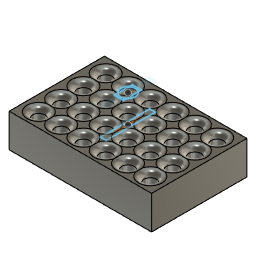
simple_rack v2 (Autodesk Fusion 360 design; units mm, degrees)
Autodesk Fusion 360 part; units mm, degrees
note: some values were not read from the file. Chosen so that the rebuilt part matches the saved one: which face or edge a step refers to. Set by a fixed rule: which sketch regions a step uses.
sketch "Sketch1" plane through (0, 0, 0) normal (0, 0, 1) x (1, 0, 0)
  circle A0 centre (0, 0) radius 5.5
  circle A1 centre (0, 0) radius 7
  circle A2 centre (20, 0) radius 7
  circle A3 centre (20, 0) radius 5.5
  circle A4 centre (40, 0) radius 7
  circle A5 centre (40, 0) radius 5.5
  circle A6 centre (60, 0) radius 7
  circle A7 centre (60, 0) radius 5.5
  circle A8 centre (80, 0) radius 7
  circle A9 centre (80, 0) radius 5.5
  circle A10 centre (100, 0) radius 7
  circle A11 centre (100, 0) radius 5.5
  circle A12 centre (0, 20) radius 7
  circle A13 centre (0, 20) radius 5.5
  circle A14 centre (20, 20) radius 7
  circle A15 centre (20, 20) radius 5.5
  circle A16 centre (40, 20) radius 7
  circle A17 centre (40, 20) radius 5.5
  circle A18 centre (60, 20) radius 7
  circle A19 centre (60, 20) radius 5.5
  circle A20 centre (80, 20) radius 7
  circle A21 centre (80, 20) radius 5.5
  circle A22 centre (100, 20) radius 7
  circle A23 centre (100, 20) radius 5.5
  circle A24 centre (0, 40) radius 7
  circle A25 centre (0, 40) radius 5.5
  circle A26 centre (20, 40) radius 7
  circle A27 centre (20, 40) radius 5.5
  circle A28 centre (40, 40) radius 7
  circle A29 centre (40, 40) radius 5.5
  circle A30 centre (60, 40) radius 7
  circle A31 centre (60, 40) radius 5.5
  circle A32 centre (80, 40) radius 7
  circle A33 centre (80, 40) radius 5.5
  circle A34 centre (100, 40) radius 7
  circle A35 centre (100, 40) radius 5.5
  circle A36 centre (0, 60) radius 7
  circle A37 centre (0, 60) radius 5.5
  circle A38 centre (20, 60) radius 7
  circle A39 centre (20, 60) radius 5.5
  circle A40 centre (40, 60) radius 7
  circle A41 centre (40, 60) radius 5.5
  circle A42 centre (60, 60) radius 7
  circle A43 centre (60, 60) radius 5.5
  circle A44 centre (80, 60) radius 7
  circle A45 centre (80, 60) radius 5.5
  circle A46 centre (100, 60) radius 7
  circle A47 centre (100, 60) radius 5.5
  line L0 (-13.88, -12.74) -> (113.88, -12.74)
  line L1 (113.88, -12.74) -> (113.88, 72.74)
  line L2 (113.88, 72.74) -> (-13.88, 72.74)
  line L3 (-13.88, 72.74) -> (-13.88, -12.74)
  line L4 (20, 60) -> (20, 72.74)
  line L5 (20, 0) -> (20, -12.74)
  line L6 (-13.88, 40) -> (0, 40)
  line L7 (100, 40) -> (113.88, 40)
  circle A48 centre (0, 0) radius 4.2426
  circle A49 centre (20, 0) radius 4.2426
  circle A50 centre (40, 0) radius 4.2426
  circle A51 centre (60, 0) radius 4.2426
  circle A52 centre (80, 0) radius 4.2426
  circle A53 centre (100, 0) radius 4.2426
  circle A54 centre (0, 20) radius 4.2426
  circle A55 centre (20, 20) radius 4.2426
  circle A56 centre (40, 20) radius 4.2426
  circle A57 centre (60, 20) radius 4.2426
  circle A58 centre (80, 20) radius 4.2426
  circle A59 centre (100, 20) radius 4.2426
  circle A60 centre (0, 40) radius 4.2426
  circle A61 centre (20, 40) radius 4.2426
  circle A62 centre (40, 40) radius 4.2426
  circle A63 centre (60, 40) radius 4.2426
  circle A64 centre (80, 40) radius 4.2426
  circle A65 centre (100, 40) radius 4.2426
  circle A66 centre (0, 60) radius 4.2426
  circle A67 centre (20, 60) radius 4.2426
  circle A68 centre (40, 60) radius 4.2426
  circle A69 centre (60, 60) radius 4.2426
  circle A70 centre (80, 60) radius 4.2426
  circle A71 centre (100, 60) radius 4.2426
  dimension "d1" = 11
  dimension "d2" = 14
  dimension "d5" = 20
  dimension "d6" = 20
  dimension "d7" = 127.76
  dimension "d8" = 85.48
  constraint coincident A0.centre A1.centre
  constraint concentric A0 A1
  constraint horizontal L0
  constraint vertical L1
  constraint horizontal L2
  constraint vertical L3
  constraint coincident A38.centre A39.centre
  constraint coincident L2 L4.end
  constraint perpendicular L2 L4
  constraint coincident A2.centre A3.centre
  constraint coincident L0 L5.end
  constraint perpendicular L0 L5
  constraint coincident L3 L6.start
  constraint coincident A24.centre A25.centre
  constraint perpendicular L3 L6
  constraint coincident A34.centre A35.centre
  constraint coincident L1 L7.end
  constraint perpendicular L1 L7
  constraint equal L6 L7
  constraint equal L4 L5
  constraint concentric A0 A48
  measures "d1" diameter of A0
  measures "d2" diameter of A1
  measures "d7" distance of L1.end L2.end
  measures "d8" distance of L0.start L2.end
extrude "Extrude2" add sketch "Sketch1" along normal blind 30 contours A1 | A2 | A4 | A6 | A8 | A10 | A12 | A14 | A16 | A18 | A20 | A22 | A24 | A26 | A28 | A30 | A32 | A34 | A36 | A38 | A40 | A42 | A44 | A46 | L0 L1 L2 L3
fillet "Fillet2" radius 5 24 edges at (94.8722, 61.9889, 30) (74.8722, 61.9889, 30) (54.8722, 61.9889, 30) (34.8722, 61.9889, 30) (14.8722, 61.9889, 30) (-5.1278, 61.9889, 30) (-5.1278, 41.9889, 30) (14.8722, 41.9889, 30) (34.8722, 41.9889, 30) (54.8722, 41.9889, 30) (74.8722, 41.9889, 30) (94.8722, 41.9889, 30) (94.8722, 21.9889, 30) (74.8722, 21.9889, 30) (54.8722, 21.9889, 30) (34.8722, 21.9889, 30) (14.8722, 21.9889, 30) (-5.1278, 21.9889, 30) (-5.1278, 1.9889, 30) (14.8722, 1.9889, 30) (34.8722, 1.9889, 30) (54.8722, 1.9889, 30) (74.8722, 1.9889, 30) (94.8722, 1.9889, 30)
extrude "Extrude3" add sketch "Sketch1" along normal blind 1 contours A0 | A3 | A5 | A7 | A9 | A11 | A13 | A15 | A17 | A19 | A21 | A23 | A25 | A27 | A29 | A31 | A33 | A35 | A37 | A39 | A41 | A43 | A45 | A47
sketch "Sketch2" plane through (0, 0, 30) normal (0, 0, 1) x (-1, 0, 0)
  arc A0 (-50, -23.2016) -> (-43.2016, -30) centre (-40, -20) ccw
  arc A1 (-56.7984, -30) -> (-50, -23.2016) centre (-60, -20) ccw
  arc A2 (-50, -36.7984) -> (-56.7984, -30) centre (-60, -40) ccw
  arc A3 (-43.2016, -30) -> (-50, -36.7984) centre (-40, -40) ccw
  line L0 (-52.5, -8) -> (-47.5, -8)
  line L1 (-47.5, -8) -> (-47.5, -52)
  line L2 (-47.5, -52) -> (-52.5, -52)
  line L3 (-52.5, -52) -> (-52.5, -8)
  line L4 (-52.5, -8) -> (-47.5, -52) construction
  line L5 (-47.5, -8) -> (-52.5, -52) construction
  point P0 (-50, -30)
  dimension "d17" = 5
  constraint horizontal L0
  constraint perpendicular L0 L1
  constraint parallel L0 L2
  constraint parallel L1 L3
  constraint coincident L4 P0
  constraint coincident L5 P0
  measures "d17" distance of L1.end L2.end
sketch "Sketch3" plane through (0, 0, 55) normal (0, 0, 1) x (-1, 0, 0)
  line L0 (-52.5, -52) -> (-47.5, -52)
  line L1 (-47.5, -52) -> (-47.5, -8)
  line L2 (-47.5, -8) -> (-52.5, -8)
  line L3 (-52.5, -8) -> (-52.5, -52)
  circle A0 centre (-50, -30) radius 6.5
  line L4 (-54, -22) -> (-46, -22)
  line L5 (-46, -22) -> (-46, -38)
  line L6 (-46, -38) -> (-54, -38)
  line L7 (-54, -38) -> (-54, -22)
  line L8 (-54, -22) -> (-46, -38) construction
  line L9 (-46, -22) -> (-54, -38) construction
  point P0 (-50, -30)
  dimension "d20" = 13
  constraint horizontal L4
  constraint perpendicular L4 L5
  constraint parallel L4 L6
  constraint parallel L5 L7
  constraint coincident L8 P0
  constraint coincident L9 P0
  constraint coincident P0 A0.centre
  measures "d20" diameter of A0
sketch "Sketch4" plane through (0, 0, -10) normal (0, 0, -1) x (1, 0, 0)
  circle A0 centre (100, -40) radius 9.6
  circle A1 centre (80, -60) radius 9.6
  circle A2 centre (60, -60) radius 9.6
  circle A3 centre (40, -40) radius 9.6
  circle A4 centre (20, -60) radius 9.6
  circle A5 centre (0, -40) radius 9.6
  circle A6 centre (20, -20) radius 9.6
  circle A7 centre (60, -20) radius 9.6
  circle A8 centre (100, -20) radius 9.6
  circle A9 centre (80, 0) radius 9.6
  circle A10 centre (40, 0) radius 9.6
  circle A11 centre (20, 0) radius 9.6
  line L0 (-13.88, 12.74) -> (-13.88, -72.74)
  line L1 (-13.88, -72.74) -> (113.88, -72.74)
  line L2 (113.88, -72.74) -> (113.88, 12.74)
  line L3 (113.88, 12.74) -> (-13.88, 12.74)
  circle A12 centre (0, 0) radius 9.6
  circle A13 centre (60, 0) radius 9.6
  circle A14 centre (100, 0) radius 9.6
  circle A15 centre (80, -20) radius 9.6
  circle A16 centre (40, -20) radius 9.6
  circle A17 centre (0, -20) radius 9.6
  circle A18 centre (0, -60) radius 9.6
  circle A19 centre (20, -40) radius 9.6
  circle A20 centre (40, -60) radius 9.6
  circle A21 centre (60, -40) radius 9.6
  circle A22 centre (80, -40) radius 9.6
  circle A23 centre (100, -60) radius 9.6
  line L4 (55, -55) -> (45, -55)
  line L5 (45, -55) -> (45, -5)
  line L6 (45, -5) -> (55, -5)
  line L7 (55, -5) -> (55, -55)
  line L8 (55, -55) -> (45, -5) construction
  line L9 (45, -55) -> (55, -5) construction
  point P0 (50, -30)
  constraint horizontal L4
  constraint perpendicular L4 L5
  constraint parallel L4 L6
  constraint parallel L5 L7
  constraint coincident L8 P0
  constraint coincident L9 P0
extrude "Extrude9" add sketch "Sketch1" along normal blind 1 contours A48 | A49 | A50 | A51 | A52 | A53 | A54 | A55 | A56 | A57 | A58 | A59 | A60 | A61 | A62 | A63 | A64 | A65 | A66 | A67 | A68 | A69 | A70 | A71
